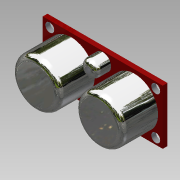
# Autodesk Inventor part: srf08
Saved by Autodesk Inventor 2015 SP1 (Build 190203100, 203)
## iProperties
Created: 2015-01-28
Part Number: srf08
Material: Generic
Document SubType Name: Modeling
Designer: Rafi Kurnia Putra
Density: 1 g/cm^3
Appearance: Default
Mass: 6.86402 g
Surface Area: 32.9466 cm^2
Volume: 6.86402 cm^3
Author: Rafi Kurnia Putra
Autodesk Inventor part; units mm, degrees
ref_plane "YZ Plane" through (0, 0, 0) normal (1, 0, 0) x (0, 1, 0)
ref_plane "XZ Plane" through (0, 0, 0) normal (0, 1, 0) x (-1, 0, 0)
ref_plane "XY Plane" through (0, 0, 0) normal (0, 0, 1) x (1, 0, 0)
sketch "Sketch1" plane through (0, 0, 0) normal (0, 1, 0) x (-1, 0, 0)
  line L0 (21.605, -9.85) -> (-21.605, -9.85)
  line L1 (-21.605, -9.85) -> (-21.605, 9.85)
  line L2 (-21.605, 9.85) -> (21.605, 9.85)
  line L3 (21.605, 9.85) -> (21.605, -9.85)
  line L4 (21.605, -9.85) -> (-21.605, 9.85) construction
  line L5 (-21.605, -9.85) -> (21.605, 9.85) construction
  circle A0 centre (-19.084, -7.654) radius 1.6
  circle A1 centre (19.084, 7.654) radius 1.6
  circle A2 centre (-11.43, 0) radius 8.5
  circle A3 centre (11.43, 0) radius 8.5
  circle A4 centre (0, -6.54) radius 3
  circle A5 centre (0, 7.874) radius 0.635
  circle A6 centre (-2.54, 7.874) radius 0.635
  circle A7 centre (-5.08, 7.874) radius 0.635
  circle A8 centre (2.54, 7.874) radius 0.635
  circle A9 centre (5.08, 7.874) radius 0.635
  line L6 (0, -13) -> (0, -21) construction
  line L7 (0, -13) -> (8, -13) construction
  circle A10 centre (-19.084, 7.654) radius 1.6
  circle A11 centre (19.084, -7.654) radius 1.6
  line L8 (-25, 0) -> (-35, 0) construction
  line L9 (-25, 0) -> (-15, 0) construction
  circle A12 centre (0, 6.54) radius 3
  point P0 (0, 0)
  dimension "d0" = 43.21
  dimension "d1" = 19.7
  dimension "d2" = 3.2
  dimension "d5" = 3.2
  dimension "d8" = 17
  dimension "d9" = 17
  dimension "d14" = 6
  dimension "d26" = 1.27
  dimension "d27" = 1.27
  dimension "d28" = 1.27
  dimension "d29" = 1.27
  dimension "d30" = 1.27
  dimension "d31" = 2.54
  dimension "d32" = 2.54
  dimension "d33" = 2.54
  dimension "d34" = 2.54
  dimension "d41" = 22.86
  dimension "d43" = 10.175
  dimension "d44" = 10.175
  dimension "d45" = 6.54
  dimension "d47" = 7.874
  dimension "d48" = 7.654
  dimension "d49" = 7.654
  dimension "d50" = 7.654
  dimension "d51" = 7.654
  dimension "d52" = 90
  dimension "d53" = 180
  constraints: 20 end point, 13 centre point, 3 horizontal, 3 symmetric about line, 2 equal length, 2 midpoint, 2 parallel, 1 perpendicular, 3 other
  measures "d0" distance of L1.end L2.end
  measures "d1" distance of L0.end L1.end
  measures "d2" diameter of A0
  measures "d5" diameter of A1
  measures "d8" diameter of A2
  measures "d9" diameter of A3
  measures "d14" diameter of A4
  measures "d26" diameter of A5
  measures "d27" diameter of A6
  measures "d28" diameter of A7
  measures "d29" diameter of A8
  measures "d30" diameter of A9
  measures "d31" distance of A6.centre A5.centre
  measures "d32" distance of A7.centre A6.centre
  measures "d33" distance of A8.centre A5.centre
  measures "d34" distance of A9.centre A8.centre
  measures "d41" distance of A2.centre A3.centre
  measures "d43" distance from line of L1 A2.centre
  measures "d44" distance from line of A3.centre L3
  measures "d45" vertical distance of A4.centre A3.centre
  measures "d47" vertical distance of A3.centre A5.centre
  measures "d48" horizontal distance of A3.centre A1.centre
  measures "d49" horizontal distance of A0.centre A2.centre
  measures "d50" horizontal distance of A3.centre A1.centre
  measures "d51" horizontal distance of A2.centre A0.centre
  measures "d52" angle of L6 L7
  measures "d53" angle of L8 L9
extrude "Extrusion1" add sketch "Sketch1" along normal blind 1.7 contours L0 L1 L2 L3 | A5 | A6 A12 | A6 A12 A8 | A12 A6 | A12 A8 | A8 A12 | A7 | A9 | A10 | A11
extrude "Extrusion2" add sketch "Sketch1" along normal blind 14.6 contours A2 | A3
extrude "Extrusion3" add sketch "Sketch1" along normal blind 7.07 contours A4
sketch "Sketch2" plane through (0, 0, 0) normal (0, -1, 0) x (1, 0, 0)
  line L0 (13.454, 4.1484) -> (8.254, 4.1484)
  line L1 (8.254, 4.1484) -> (8.254, -5.9816)
  line L2 (8.254, -5.9816) -> (13.454, -5.9816)
  line L3 (13.454, -5.9816) -> (13.454, 4.1484)
  line L4 (13.454, 4.1484) -> (8.254, -5.9816) construction
  line L5 (8.254, 4.1484) -> (13.454, -5.9816) construction
  point P0 (0, 0)
  point P1 (10.854, -0.9166)
  dimension "d22" = 5.2
  dimension "d23" = 10.13
  constraints: 12 end point, 2 midpoint, 2 parallel, 1 horizontal, 1 perpendicular
  measures "d22" distance of L2.end L1.end
  measures "d23" distance of L1.end L0.end
extrude "Extrusion4" add sketch "Sketch2" along normal blind 2
extrude "Extrusion5" cut sketch "Sketch1" along normal through all contours A5 | A6 A12 | A12 A6 | A12 A8 | A8 A12 | A7 | A9
fillet "Fillet1" radius 2 2 edges at (19.93, 14.6, 0) (-2.93, 14.6, 0)
fillet "Fillet2" radius 2 1 edges at (3, 7.07, -6.54)
extrude "Extrusion6" cut sketch "Sketch1" along normal through all contours A10 | A11
sketch "Sketch3" plane through (0, 0, 0) normal (0, -1, 0) x (1, 0, 0)
  circle A0 centre (0, 6.54) radius 3 projected
  point P0 (0, 0)
body "Solid1"
